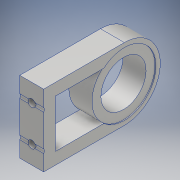
# Autodesk Inventor part: 베어링받침대
Saved by Autodesk Inventor 2017 (Build 210142000, 142)
## iProperties
Part Number: 베어링받침대
Material: 알루미늄 6061
Document SubType Name: Modeling
Designer: minom
Density: 2.7 g/cm^3
Appearance: 알루미늄 - 평지
Mass: 10.1645 g
Surface Area: 28.3876 cm^2
Volume: 3.76464 cm^3
Author: minom
Autodesk Inventor part; units mm, degrees
ref_plane "YZ Plane" through (0, 0, 0) normal (1, 0, 0) x (0, 1, 0)
ref_plane "XZ Plane" through (0, 0, 0) normal (0, 1, 0) x (-1, 0, 0)
ref_plane "XY Plane" through (0, 0, 0) normal (0, 0, 1) x (1, 0, 0)
sketch "스케치1" plane through (0, 0, 0) normal (1, 0, 0) x (0, 1, 0)
  line L0 (0, 0) -> (27, 0)
  line L1 (27, -24) -> (0, -24)
  line L2 (0, -24) -> (0, 0)
  circle A0 centre (27, -12) radius 7.55
  arc A1 (27, -24) -> (27, 0) centre (27, -12) ccw
  dimension "d2" = 15.1
  dimension "d3" = 12
  dimension "d4" = 27
  dimension "d8" = 24
  constraints: 6 end point, 2 centre point, 2 point on circle, 1 coincident, 1 horizontal, 1 parallel, 1 tangent
  measures "d2" diameter of A0
  measures "d3" distance from line of L1 A0.centre
  measures "d4" distance from line of L2 A0.centre
  measures "d8" distance between parallel lines of L1 L0
extrude "돌출2" add sketch "스케치1" along normal blind 8
sketch "스케치2" plane through (8, 0, 0) normal (1, 0, 0) x (0, 0, -1)
  circle A0 centre (12, 27) radius 7.55 projected
  line L0 (0, 27) -> (0, 0) projected
  line L1 (0, 0) -> (24, 0) projected
  line L2 (24, 0) -> (24, 27) projected
  arc A1 (24, 27) -> (0, 27) centre (12, 27) ccw projected
  arc A2 (4, 20.1223) -> (20, 20.1223) centre (12, 27) ccw
  line L3 (4, 4) -> (4, 20.1223)
  line L4 (20, 20.1223) -> (20, 4)
  line L5 (20, 4) -> (4, 4)
  dimension "d12" = 3
  dimension "d13" = 4
  constraints: 6 end point, 2 point on circle, 1 centre point
  measures "d12" radial gap between concentric circles of A0 A2
  measures "d13" distance between parallel lines of L3 L0
extrude "돌출3" cut sketch "스케치2" against normal blind 8 contours A2 L4 L5 L3
sketch "스케치3" plane through (0, 0, -24) normal (0, -1, 0) x (1, 0, 0)
  circle A0 centre (4, 18) radius 1.25
  circle A1 centre (4, 6) radius 1.25
  line L0 (8, 24) -> (8, 0) projected
  line L1 (0, 24) -> (8, 24) projected
  line L2 (0, 0) -> (8, 0) projected
  dimension "d16" = 2.5
  dimension "d17" = 2.5
  dimension "d18" = 4
  dimension "d19" = 4
  dimension "d20" = 6
  dimension "d21" = 6
  constraints: 2 centre point
  measures "d16" diameter of A0
  measures "d17" diameter of A1
  measures "d18" distance from line of A0.centre L0
  measures "d19" distance from line of A1.centre L0
  measures "d20" distance from line of A0.centre L1
  measures "d21" distance from line of A1.centre L2
extrude "돌출4" cut sketch "스케치3" against normal blind 8
sketch "스케치4" plane through (8, 0, 0) normal (1, 0, 0) x (0, 0, -1)
  line L0 (4.75, 4) -> (7.25, 4) projected
  line L1 (7.25, 0) -> (4.75, 0) projected
  line L2 (16.75, 4) -> (19.25, 4) projected
  line L3 (19.25, 0) -> (16.75, 0) projected
  arc A0 (6.6614, 0) -> (5.3386, 0) centre (6, -0.75) ccw
  arc A1 (18.6614, 0) -> (17.3386, 0) centre (18, -0.75) ccw
  line L4 (0, 0) -> (24, 0) projected
  dimension "d24" = 2
  dimension "d25" = 2
  constraints: 4 point on circle, 2 centre point, 5 other
  measures "d24" diameter of A0
  measures "d25" diameter of A1
extrude "돌출5" cut sketch "스케치4" against normal blind 8
sketch "스케치5" plane through (8, 0, 0) normal (1, 0, 0) x (0, 0, -1)
  arc A0 (6.6614, 0) -> (5.3386, 0) centre (6, -0.75) ccw projected
  line L0 (6.6614, 0) -> (17.3386, 0) projected
  arc A1 (18.6614, 0) -> (17.3386, 0) centre (18, -0.75) ccw projected
  line L1 (18.6614, 0) -> (24, 0) projected
  line L2 (24, 0) -> (24, 27) projected
  arc A2 (24, 27) -> (0, 27) centre (12, 27) ccw projected
  line L3 (0, 27) -> (0, 0) projected
  line L4 (0, 0) -> (5.3386, 0) projected
  circle A3 centre (12, 27) radius 7.55 projected
  line L5 (20, 4) -> (4, 4) projected
  line L6 (4, 4) -> (4, 20.1223) projected
  arc A4 (4, 20.1223) -> (20, 20.1223) centre (12, 27) ccw projected
  line L7 (20, 20.1223) -> (20, 4) projected
  circle A5 centre (12, 27) radius 10.55
  constraints: 1 centre point, 1 coincident, 1 concentric
extrude "돌출6" cut sketch "스케치5" against normal blind 0.3 contours A4 A5
